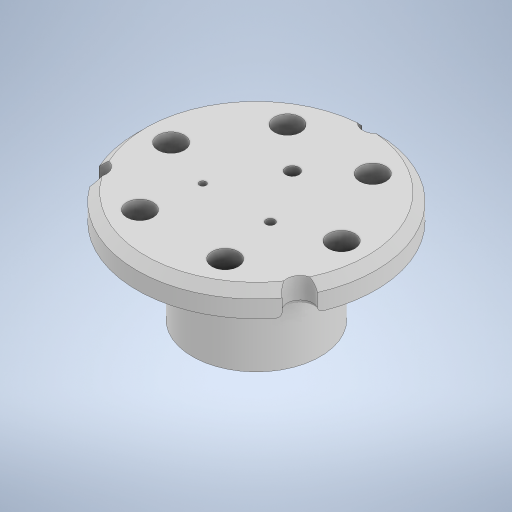
# Autodesk Inventor part: Schneidtrommel
Saved by Autodesk Inventor 2024 (Build 280153000, 153)
## iProperties
Created: 2023-05-12
Part Number: Schneidtrommel
Material: Generic
Document SubType Name: Modeling
Designer: Raj
Density: 1 g/cm^3
Appearance: Default
Author: Raj
Autodesk Inventor part; units mm, degrees
ref_plane "YZ Plane" through (0, 0, 0) normal (1, 0, 0) x (0, 1, 0)
ref_plane "XZ Plane" through (0, 0, 0) normal (0, 1, 0) x (-1, 0, 0)
ref_plane "XY Plane" through (0, 0, 0) normal (0, 0, 1) x (1, 0, 0)
sketch "Sketch1" plane through (0, 0, 0) normal (0, 0, 1) x (1, 0, 0)
  circle A0 centre (0, 0) radius 28
  circle A1 centre (-20, 0) radius 3.1
  circle A2 centre (-10, -17.3205) radius 3.1
  circle A3 centre (10, -17.3205) radius 3.1
  circle A4 centre (20, 0) radius 3.1
  circle A5 centre (10, 17.3205) radius 3.1
  circle A6 centre (-10, 17.3205) radius 3.1
  dimension "d0" = 56
  dimension "d1" = 6.2
  dimension "d2" = 20
  dimension "d3" = 0
  dimension "d6" = 360
  constraints: 7 centre point, 1 coincident, 13 other
  measures "d0" diameter of A0
  measures "d1" diameter of A1
  measures "d2" distance of A1.centre point (0, 0)
  measures "d3" vertical distance of A1.centre point (0, 0)
extrude "Extrusion1" add sketch "Sketch1" along normal blind 6
sketch "Sketch2" plane through (0, 0, 0) normal (0, 0, -1) x (-1, 0, 0)
  circle A0 centre (0, 0) radius 15
  dimension "d10" = 30
  constraints: 1 centre point, 1 coincident
  measures "d10" diameter of A0
extrude "Extrusion2" add sketch "Sketch2" along normal blind 20
sketch "Sketch3" plane through (0, 0, 6) normal (0, 0, 1) x (1, 0, 0)
  circle A0 centre (0, 0) radius 28 projected
  circle A1 centre (0, 28) radius 3.05
  circle A2 centre (-24.2487, -14) radius 3.05
  circle A3 centre (24.2487, -14) radius 3.05
  circle A4 centre (0, 8.45) radius 1.55
  line L0 (0, 28) -> (0, 0) construction
  line L1 (0, 0) -> (24.2487, -14) construction
  line L2 (-24.2487, -14) -> (0, 0) construction
  circle A5 centre (7.7509, -4.475) radius 1.05
  circle A6 centre (-7.9674, -4.6) radius 0.8
  circle A7 centre (0, 0) radius 10 construction
  point P0 (25.6276, -11.2795)
  point P1 (22.5821, -16.5544)
  point P2 (-25.6276, -11.2795)
  point P3 (-22.5821, -16.5544)
  point P4 (-3.0455, 27.8339)
  point P5 (3.0455, 27.8339)
  dimension "d13" = 6.1
  dimension "d17" = 360
  dimension "d19" = 3.1
  dimension "d20" = 0
  dimension "d21" = 0
  dimension "d22" = 2.1
  dimension "d23" = 1.6
  dimension "d24" = 20
  constraints: 7 centre point, 6 end point, 3 tangent, 2 point on line, 1 coincident, 9 other
  measures "d13" diameter of A1
  measures "d19" diameter of A4
  measures "d20" horizontal distance of point (0, 0) L0.start
  measures "d21" distance from line of A4.centre L0
  measures "d22" diameter of A5
  measures "d23" diameter of A6
  measures "d24" diameter of A7
extrude "Extrusion3" cut sketch "Sketch3" against normal through all contours A1 A0 | A0 A3 | A2 A0 | A4 | A5 | A6 picked at (0.1183, 26.9779) picked at (23.3044, -13.5914) picked at (-23.3241, -13.5486)
chamfer "Chamfer1" distance 2 angle 45 3 edges at (-24.2487, 14, 6) (0, -28, 6) (24.2487, 14, 6)
fillet "Fillet1" radius 1 3 edges at (21.6073, -12.475, 0) (-21.6073, -12.475, 0) (0, 24.95, 0)
body "Solid1"
